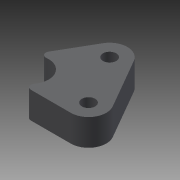
# Autodesk Inventor part: X_zaslepka
Saved by Autodesk Inventor 2013 (Build 170138000, 138)
## iProperties
Created: 2013-12-11
Part Number: X_zaslepka
Material: Generic
Document SubType Name: Modeling
Designer: dzban
Density: 1 g/cm^3
Author: dzban
Autodesk Inventor part; units mm, degrees
ref_plane "YZ Plane" through (0, 0, 0) normal (1, 0, 0) x (0, 1, 0)
ref_plane "XZ Plane" through (0, 0, 0) normal (0, 1, 0) x (-1, 0, 0)
ref_plane "XY Plane" through (0, 0, 0) normal (0, 0, 1) x (1, 0, 0)
sketch "Sketch1" plane through (0, 0, 0) normal (0, 0, 1) x (1, 0, 0)
  circle A0 centre (13, 0) radius 1.5
  circle A1 centre (6.5, 11.2583) radius 1.5
  arc A2 (9.9641, 13.2583) -> (3.0359, 13.2583) centre (6.5, 11.2583) ccw
  arc A3 (13, -4) -> (16.4641, 2) centre (13, 0) ccw
  line L0 (9.9641, 13.2583) -> (16.4641, 2)
  arc A4 (3.2, -2.4) -> (-0.4785, 3.9713) centre (0, 0) ccw
  line L1 (4, -4) -> (13, -4)
  line L2 (-1.4641, 5.4641) -> (3.0359, 13.2583)
  arc A5 (-1.4641, 5.4641) -> (-0.4785, 3.9713) centre (-0.5981, 4.9641) ccw
  arc A6 (3.2, -2.4) -> (4, -4) centre (4, -3) ccw
  point P0 (0, -4)
  point P1 (-3.4641, 2)
  dimension "d0" = 3
  dimension "d1" = 3
  dimension "d3" = 13
  dimension "d4" = 13
  dimension "d24" = 60
  dimension "d25" = 8
  dimension "d26" = 8
  dimension "d27" = 8
  dimension "d30" = 1
  constraints: 12 point on circle, 10 tangent, 7 centre point, 6 end point, 4 coincident, 2 horizontal alignment, 2 point on line, 1 equal radius
  measures "d0" diameter of A1
  measures "d1" diameter of A0
  measures "d3" distance of point (0, 0) A0.centre
  measures "d4" distance of point (0, 0) A1.centre
  measures "d25" diameter of A2
  measures "d26" diameter of A3
  measures "d27" diameter of A4
  measures "d30" radius of A5
extrude "Extrusion1" add sketch "Sketch1" along normal blind 6
body "Solid1"
